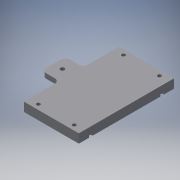
# Autodesk Inventor part: PRING_piston_case_half
Saved by Autodesk Inventor 2018 (Build 220112000, 112)
## iProperties
Created: 2026-05-31
Part Number: PRING_piston_case_half
Material: Generic
Document SubType Name: Modeling
Designer: neo
Density: 1 g/cm^3
Appearance: Default
Author: neo
Autodesk Inventor part; units mm, degrees
ref_plane "YZ Plane" through (0, 0, 0) normal (1, 0, 0) x (0, 1, 0)
ref_plane "XZ Plane" through (0, 0, 0) normal (0, 1, 0) x (-1, 0, 0)
sketch "Sketch1" plane through (0, 0, 0) normal (1, 0, 0) x (0, 1, 0)
  line L0 (-1.5973, 19.3351) -> (-9.0973, 19.3351)
  line L1 (-9.0973, -60.6649) -> (-1.5973, -60.6649)
  line L2 (-1.5973, -60.6649) -> (-1.5973, 19.3351)
  line L3 (20.1932, -20.6649) -> (-21.0203, -20.6649)
  line L4 (-9.0973, 19.3351) -> (-9.0973, -15.5649)
  line L5 (-9.0973, -25.7649) -> (-9.0973, -60.6649)
  circle A0 centre (-9.0973, -20.6649) radius 5.1 construction
  line L6 (-11.2098, -15.5649) -> (-6.9848, -15.5649)
  line L7 (-6.9848, -15.5649) -> (-3.9973, -18.5524)
  line L8 (-3.9973, -18.5524) -> (-3.9973, -22.7774)
  line L9 (-3.9973, -22.7774) -> (-6.9848, -25.7649)
  line L10 (-6.9848, -25.7649) -> (-11.2098, -25.7649)
  line L11 (-10.6473, 10.8851) -> (-7.5473, 10.8851)
  line L12 (-7.5473, 10.8851) -> (-7.5473, 7.7851)
  line L13 (-7.5473, 7.7851) -> (-10.6473, 7.7851)
  line L14 (-10.6473, 7.7851) -> (-10.6473, 10.8851)
  line L15 (-10.6473, 10.8851) -> (-7.5473, 7.7851) construction
  line L16 (-7.5473, 10.8851) -> (-10.6473, 7.7851) construction
  point P0 (0, 0)
  point P1 (-9.0973, 9.3351)
  dimension "d6" = 10.2
  dimension "d2" = 7.5
  dimension "d3" = 80
  dimension "d7" = 3.1
  dimension "d9" = 60
  constraints: 34 end point, 5 parallel, 4 horizontal, 4 midpoint, 4 perpendicular, 2 point on line, 1 coincident, 1 vertical alignment, 13 other
  measures "d2" distance between parallel lines of L2 L4
  measures "d3" distance between parallel lines of L1 L0
  measures "d7" distance of L11.end L12.end
  measures "d9" diameter of point (-9.097, 9.335) L3
extrude "Extrusion1" add sketch "Sketch1" along normal blind 46.2 contours L2 L3 L8 L7 L6 L4 L13 L12 L11 L0 | L2 L1 L5 L10 L9 L8 L3 | L11 L12 L13 L4
extrude "Extrusion2" cut sketch "Sketch1" along normal through all contours L11 L12 L13 L4 | L4 L13 L14 L11
ref_plane "Work Plane1" through (0, -1.5973, -20.6649) normal (0, 0, 1) x (1, 0, 0)
mirror "Mirror1" about plane through (0, -1.5973, -20.6649) normal (0, 0, 1) of "Extrusion2"
sketch "Sketch2" plane through (0, -9.0973, 19.3351) normal (0, -1, 0) x (1, 0, 0)
  line L0 (0, 0) -> (0, -8.45) projected
  line L1 (0, -4.225) -> (55.9081, -4.225)
  line L2 (0, 0) -> (46.2, 0) projected
  line L3 (23.1, 0) -> (23.1, -31.5844)
  line L4 (8, 4.0283) -> (8, -8.7646)
  circle A0 centre (8, -4.225) radius 1.5
  circle A1 centre (38.2, -4.225) radius 1.5
  point P0 (0, -19.3351)
  dimension "d12" = 8
  dimension "d13" = 3
  constraints: 6 end point, 2 centre point, 2 midpoint, 2 point on line, 2 vertical, 1 horizontal, 1 symmetric about line, 1 other
  measures "d12" distance between parallel lines of L0 L4
  measures "d13" diameter of A0
extrude "Extrusion3" cut sketch "Sketch2" against normal through all contours A1 L1 | L1 A1 | A0 L4 L1 | L1 L4 A0 | A0 L1 L4 | L1 A0 L4
mirror "Mirror2" about plane through (0, -1.5973, -20.6649) normal (0, 0, 1) of "Extrusion3"
sketch "Sketch3" plane through (0, -9.0973, 19.3351) normal (0, -1, 0) x (1, 0, 0)
  line L0 (0, -68.45) -> (46.2, -68.45) projected
  line L1 (46.2, -34.9) -> (43.2, -34.9)
  line L2 (43.2, -34.9) -> (43.2, -68.45)
  line L3 (43.2, -68.45) -> (46.2, -68.45)
  line L4 (46.2, -68.45) -> (46.2, -34.9)
  line L5 (0, -34.9) -> (3, -34.9)
  line L6 (3, -34.9) -> (3, -45.1)
  line L7 (3, -45.1) -> (0, -45.1)
  line L8 (0, -45.1) -> (0, -34.9)
  point P0 (0, -19.3351)
  dimension "d16" = 3
  dimension "d17" = 3
  constraints: 16 end point, 4 parallel, 2 horizontal, 2 perpendicular, 1 point on line
  measures "d16" distance between parallel lines of L8 L6
  measures "d17" distance between parallel lines of L4 L2
extrude "Extrusion4" add sketch "Sketch3" against normal through all
sketch "Sketch4" plane through (0, -1.5973, -60.6649) normal (0, 1, 0) x (1, 0, 0)
  line L0 (0, -50) -> (-15, -50)
  line L1 (-15, -50) -> (-15, -30)
  line L2 (-15, -30) -> (0, -30)
  line L3 (0, -30) -> (0, -50)
  line L4 (58.44, -40) -> (-27.24, -40) projected
  line L5 (0, 0) -> (0, -80) construction
  circle A0 centre (-7.5, -40) radius 1.75
  point P0 (0, -60.6649)
  dimension "d20" = 15
  dimension "d21" = 20
  dimension "d22" = 3.5
  dimension "d23" = 7.5
  constraints: 8 end point, 2 parallel, 1 centre point, 1 collinear, 1 horizontal, 1 perpendicular, 1 point on line, 1 other
  measures "d20" distance between parallel lines of L3 L1
  measures "d21" distance of L0.end L1.end
  measures "d22" diameter of A0
  measures "d23" distance from line of L1 A0.centre
extrude "Extrusion5" add sketch "Sketch4" against normal blind 4 contours L0 L1 L4 A0 L3 | L4 A0 L1 L2 L3
fillet "Fillet1" radius 4 4 edges at (0, -3.5973, -10.6649) (-15, -3.5973, -10.6649) (-15, -3.5973, -30.6649) (0, -3.5973, -30.6649)
equation "\"d17\" = d16"
body "Solid1"
